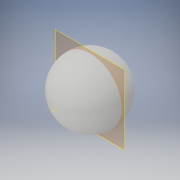
# Autodesk Inventor part: ball
Saved by Autodesk Inventor 2019 (Build 230136000, 136)
## iProperties
Created: 2018-07-14
Part Number: ball
Material: Generic
Document SubType Name: Modeling
Designer: steele
Density: 1 g/cm^3
Appearance: Default
Author: steele
Autodesk Inventor part; units mm, degrees
ref_plane "YZ Plane" through (0, 0, 0) normal (1, 0, 0) x (0, 1, 0)
ref_plane "XZ Plane" through (0, 0, 0) normal (0, 1, 0) x (-1, 0, 0)
sketch "Sketch2" plane through (0, 0, 0) normal (0, 0, 1) x (1, 0, 0)
  arc A0 (0, -6.0325) -> (0, 6.0325) centre (0, 0) ccw
  line L0 (0, 6.0325) -> (0, -6.0325)
  dimension "d1" = 12.065
  constraints: 2 end point, 2 point on circle, 1 centre point, 1 coincident, 1 vertical
  measures "d1" diameter of A0
revolve "Revolution1" add sketch "Sketch2" angle 360 about axis through (0, 6.0325, 0) along (0, -1, 0)
equation "\"d1\" = diameterOfBall"
equation "\"allowanceForBallToRotate\" = 0.635"
equation "\"diameterOfBall\" = 12.065"
body "Solid1"
